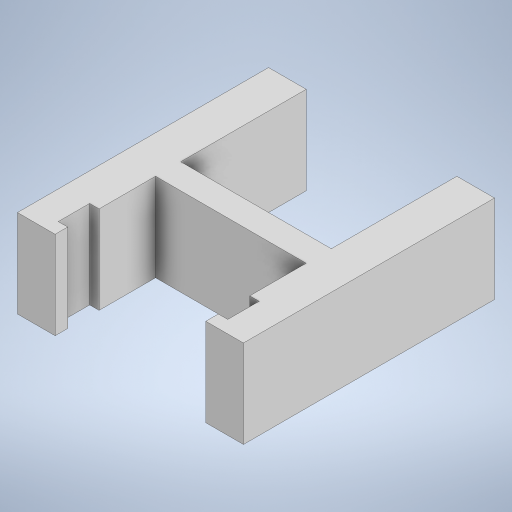
# Autodesk Inventor part: CO-1-01-stepperControllerMount
Saved by Autodesk Inventor 2024 (Build 280153000, 153)
## iProperties
Created: 2023-11-20
Part Number: CO-1-01-stepperControllerMount
Material: Generic
Document SubType Name: Modeling
Designer: t205b
Density: 1 g/cm^3
Appearance: Default
Author: t205b
Autodesk Inventor part; units mm, degrees
ref_plane "YZ Plane" through (0, 0, 0) normal (1, 0, 0) x (0, 1, 0)
ref_plane "XZ Plane" through (0, 0, 0) normal (0, 1, 0) x (-1, 0, 0)
ref_plane "XY Plane" through (0, 0, 0) normal (0, 0, 1) x (1, 0, 0)
sketch "Sketch1" plane through (0, 0, 0) normal (0, 1, 0) x (-1, 0, 0)
  line L0 (-3.0388, 7.0833) -> (-6.0388, 7.0833)
  line L1 (-6.0388, 7.0833) -> (-6.0388, -12.9167)
  line L2 (-6.0388, -12.9167) -> (-3.0388, -12.9167)
  line L3 (-3.0388, -12.9167) -> (-3.0388, -2.9167)
  line L4 (-3.0388, -2.9167) -> (8.9612, -2.9167)
  line L5 (8.9612, -12.9167) -> (11.9612, -12.9167)
  line L6 (11.9612, -12.9167) -> (11.9612, 7.0833)
  line L7 (11.9612, 7.0833) -> (8.9612, 7.0833)
  line L8 (8.9612, 7.0833) -> (8.9612, 6.0833)
  line L9 (8.9612, 6.0833) -> (9.7112, 6.0833)
  line L10 (9.7112, 6.0833) -> (9.7112, 3.5833)
  line L11 (9.7112, 3.5833) -> (8.9612, 3.5833)
  line L12 (8.9612, 3.5833) -> (8.9612, -0.9167)
  line L13 (8.9612, -0.9167) -> (-3.0388, -0.9167)
  line L14 (-3.0388, -0.9167) -> (-3.0388, 3.5833)
  line L15 (-3.7888, 3.5833) -> (-3.7888, 6.0833)
  line L16 (-3.7888, 6.0833) -> (-3.0388, 6.0833)
  line L17 (-3.0388, 3.5833) -> (-3.7888, 3.5833)
  line L18 (-3.0388, 6.0833) -> (-3.0388, 7.0833)
  line L19 (8.9612, -12.9167) -> (8.9612, -2.9167)
  point P0 (0, 0)
  dimension "d0" = 2.5
  dimension "d1" = 3
  dimension "d2" = 3
  dimension "d3" = 10
  dimension "d4" = 10
  dimension "d5" = 2
  dimension "d6" = 3
  dimension "d8" = 1
  dimension "d9" = 8
  dimension "d10" = 18
  dimension "d11" = 0.75
  dimension "d12" = 0.75
  dimension "d13" = 3
  constraints: 40 end point, 12 perpendicular, 10 point on line, 2 horizontal, 1 vertical, 1 other
  measures "d0" distance between parallel lines of L16 L17
  measures "d1" distance between parallel lines of L3 L1
  measures "d2" distance between parallel lines of L14 L1
  measures "d3" distance between parallel lines of L4 L2
  measures "d4" distance between parallel lines of L4 L5
  measures "d5" distance between parallel lines of L13 L4
  measures "d6" distance between parallel lines of L6 L12
  measures "d8" distance between parallel lines of L0 L16
  measures "d9" distance between parallel lines of L0 L13
  measures "d10" distance between parallel lines of L6 L1
  measures "d11" distance between parallel lines of L14 L15
  measures "d12" distance between parallel lines of L10 L12
  measures "d13" distance between parallel lines of L6 L19
extrude "Extrusion1" add sketch "Sketch1" along normal blind 7
equation "\"d2\" = d1"
equation "\"d4\" = d3"
equation "\"d6\" = d2"
equation "\"d12\" = d11"
equation "\"d13\" = d1"
body "Solid1"
